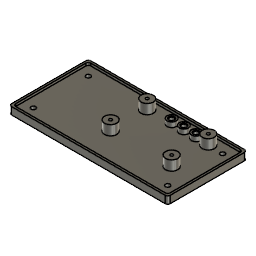
Enclosure Lid (Autodesk Fusion 360 design; units mm, degrees)
Autodesk Fusion 360 part; units mm, degrees
note: some values were not read from the file. Set by a fixed rule: the direction of a hole.
sketch "Sketch1" plane through (0, 0, 0) normal (0, 0, 1) x (1, 0, 0)
  line L0 (0, 0) -> (130, 0)
  line L1 (130, 0) -> (130, 65)
  line L2 (130, 65) -> (0, 65)
  line L3 (0, 65) -> (0, 0)
  line L4 (1.75, 1.75) -> (128.25, 1.75)
  line L5 (128.25, 1.75) -> (128.25, 63.25)
  line L6 (128.25, 63.25) -> (1.75, 63.25)
  line L7 (1.75, 63.25) -> (1.75, 1.75)
  line L8 (4, 4) -> (126, 4)
  line L9 (126, 4) -> (126, 61)
  line L10 (126, 61) -> (4, 61)
  line L11 (4, 61) -> (4, 4)
  line L12 (4, 61) -> (16, 61)
  line L13 (16, 61) -> (16, 49)
  line L14 (16, 49) -> (4, 49)
  line L15 (4, 49) -> (4, 61)
  line L16 (4, 4) -> (16, 4)
  line L17 (16, 4) -> (16, 16)
  line L18 (16, 16) -> (4, 16)
  line L19 (4, 16) -> (4, 4)
  line L20 (126, 61) -> (114, 61)
  line L21 (114, 61) -> (114, 49)
  line L22 (114, 49) -> (126, 49)
  line L23 (126, 49) -> (126, 61)
  line L24 (126, 4) -> (114, 4)
  line L25 (114, 4) -> (114, 16)
  line L26 (114, 16) -> (126, 16)
  line L27 (126, 16) -> (126, 4)
  circle A0 centre (10, 55) radius 1.75
  circle A1 centre (10, 10) radius 1.75
  circle A2 centre (120, 55) radius 1.75
  circle A3 centre (120, 10) radius 1.75
  dimension "d1" = 130
  dimension "d2" = 65
  dimension "d3" = 126.5
  dimension "d15" = 12
  dimension "d17" = 12
  dimension "d19" = 12
  dimension "d20" = 12
  dimension "d21" = 12
  dimension "d22" = 12
  dimension "d23" = 3.5
  dimension "d24" = 3.5
  dimension "d25" = 3.5
  dimension "d26" = 3.5
  dimension "d55" = 12
  dimension "d56" = 12
  dimension "d57" = 6
  dimension "d58" = 6
  dimension "d59" = 6
  dimension "d60" = 6
  dimension "d61" = 6
  dimension "d62" = 6
  dimension "d63" = 6
  dimension "d64" = 6
  dimension "d65" = 57
  dimension "d66" = 61.5
  dimension "d67" = 1.75
  dimension "d68" = 1.75
  dimension "d202" = 2.25
  dimension "d203" = 2.25
  constraint horizontal L0
  constraint vertical L1
  constraint horizontal L2
  constraint vertical L3
  constraint coincident L0.start L3.end
  constraint horizontal L4
  constraint vertical L5
  constraint horizontal L6
  constraint vertical L7
  constraint horizontal L8
  constraint vertical L9
  constraint horizontal L10
  constraint vertical L11
  constraint horizontal L12
  constraint vertical L13
  constraint horizontal L14
  constraint vertical L15
  constraint horizontal L16
  constraint vertical L17
  constraint horizontal L18
  constraint vertical L19
  constraint horizontal L20
  constraint vertical L21
  constraint horizontal L22
  constraint vertical L23
  constraint horizontal L24
  constraint vertical L25
  constraint horizontal L26
  constraint vertical L27
  measures "d1" distance of L0.start L0.end
  measures "d2" distance of L0.start L2.end
  measures "d3" distance of L4.start L4.end
  measures "d15" distance of L10.end L12.end
  measures "d17" distance of L8.start L16.end
  measures "d19" distance of L9.end L20.end
  measures "d20" distance of L9.end L22.end
  measures "d21" distance of L8.end L24.end
  measures "d22" distance of L8.end L26.end
  measures "d23" diameter of A0
  measures "d24" diameter of A1
  measures "d25" diameter of A2
  measures "d26" diameter of A3
  measures "d55" distance of L10 L14
  measures "d56" distance of L8 L18
  measures "d57" distance of L13 A0.centre
  measures "d58" distance of L10 A0.centre
  measures "d59" distance of L22 A2.centre
  measures "d60" distance of L21 A2.centre
  measures "d61" distance of L26 A3.centre
  measures "d62" distance of L25 A3.centre
  measures "d63" distance of L17 A1.centre
  measures "d64" distance of L18 A1.centre
  measures "d65" distance of L10 L16
  measures "d66" distance of L4 L6
  measures "d67" distance of L2 L6
  measures "d68" distance of L1 L5
  measures "d202" distance of L7 L11
  measures "d203" distance of L5 L23
extrude "Extrude1" add sketch "Sketch1" along normal blind 4 contours L4 L5 L6 L7 | L8 L11 L16 L17 L18 L19 | L8 L9 L10 L11 L13 L14 L17 L18 L21 L22 L25 L26 | L8 L9 L24 L25 L26 L27 | L10 L11 L12 L13 L14 L15 | L9 L10 L20 L21 L22 L23 | A0 | A1 | A2 | A3
extrude "Extrude2" add sketch "Sketch1" along normal blind 6 contours L0 L1 L2 L3
hole "Hole1" at (10, 10, 0) direction (0, 0, 1) diameter 3.75 depth 4 tip angle 118 countersink diameter 6.5 countersink angle 90
hole "Hole2" at (10, 55, 0) direction (0, 0, 1) diameter 3.75 depth 4 tip angle 118 countersink diameter 6.5 countersink angle 90
hole "Hole3" at (120, 55, 0) direction (0, 0, 1) diameter 3.75 depth 4 tip angle 118 countersink diameter 6.5 countersink angle 90
hole "Hole4" at (120, 10, 0) direction (0, 0, 1) diameter 3.75 depth 4 tip angle 118 countersink diameter 6.5 countersink angle 90
fillet "Fillet1" radius 2 1 edges at (130, 0, 3)
fillet "Fillet2" radius 2 1 edges at (1.75, 63.25, 5)
fillet "Fillet3" radius 2 1 edges at (0, 65, 3)
fillet "Fillet4" radius 2 1 edges at (128.25, 1.75, 5)
fillet "Fillet5" radius 2 1 edges at (0, 0, 3)
fillet "Fillet6" radius 2 1 edges at (128.25, 63.25, 5)
fillet "Fillet7" radius 2 1 edges at (130, 65, 3)
fillet "Fillet8" radius 2 1 edges at (1.75, 1.75, 5)
sketch "Sketch2" plane through (0, 0, 4) normal (0, 0, 1) x (-1, 0, 0)
  circle A0 centre (-120, -10) radius 1.875
  circle A1 centre (-120, -55) radius 1.875
  circle A2 centre (-10, -55) radius 1.875
  circle A3 centre (-10, -10) radius 1.875
  arc A4 (-1.75, -3.75) -> (-3.75, -1.75) centre (-3.75, -3.75) ccw
  line L0 (-3.75, -1.75) -> (-126.25, -1.75)
  arc A5 (-126.25, -1.75) -> (-128.25, -3.75) centre (-126.25, -3.75) ccw
  line L1 (-128.25, -3.75) -> (-128.25, -61.25)
  arc A6 (-128.25, -61.25) -> (-126.25, -63.25) centre (-126.25, -61.25) ccw
  line L2 (-126.25, -63.25) -> (-3.75, -63.25)
  arc A7 (-3.75, -63.25) -> (-1.75, -61.25) centre (-3.75, -61.25) ccw
  line L3 (-1.75, -61.25) -> (-1.75, -3.75)
  line L4 (-53, -60.25) -> (-113, -60.25)
  line L5 (-113, -60.25) -> (-113, -20.25)
  line L6 (-113, -20.25) -> (-53, -20.25)
  line L7 (-53, -20.25) -> (-53, -60.25)
  line L8 (-53, -50.25) -> (-53, -60.25)
  line L9 (-113, -60.25) -> (-103, -60.25)
  line L10 (-113, -50.25) -> (-113, -60.25)
  circle A8 centre (-58, -55.25) radius 1.22
  circle A9 centre (-108, -55.25) radius 1.22
  circle A10 centre (-58, -25.25) radius 1.22
  circle A11 centre (-108, -25.25) radius 1.22
  circle A12 centre (-78, -55.25) radius 1.75
  circle A13 centre (-88, -55.25) radius 1.75
  circle A14 centre (-98, -55.25) radius 1.75
  circle A15 centre (-78, -55.25) radius 3.75
  circle A16 centre (-88, -55.25) radius 3.75
  circle A17 centre (-98, -55.25) radius 3.75
  circle A18 centre (-108, -25.25) radius 5
  circle A19 centre (-58, -25.25) radius 5
  circle A20 centre (-58, -55.25) radius 5
  circle A21 centre (-108, -55.25) radius 5
  point P0 (-120, -55)
  dimension "d86" = 40
  dimension "d87" = 3
  dimension "d94" = 10
  dimension "d97" = 2.44
  dimension "d98" = 2.44
  dimension "d99" = 2.44
  dimension "d100" = 2.44
  dimension "d109" = 3.5
  dimension "d110" = 3.5
  dimension "d111" = 3.5
  dimension "d113" = 5
  dimension "d114" = 5
  dimension "d115" = 5
  dimension "d116" = 10
  dimension "d117" = 10
  dimension "d171" = 7.5
  dimension "d172" = 7.5
  dimension "d173" = 7.5
  dimension "d239" = 10
  dimension "d240" = 10
  dimension "d241" = 5
  dimension "d242" = 5
  dimension "d243" = 5
  dimension "d244" = 5
  dimension "d245" = 10
  dimension "d246" = 10
  dimension "d249" = 60
  dimension "d250" = 25
  dimension "d251" = 7
  dimension "d260" = 5
  dimension "d261" = 5
  dimension "d262" = 5
  dimension "d263" = 5
  constraint horizontal L4
  constraint vertical L5
  constraint horizontal L6
  constraint vertical L7
  constraint concentric A12 A15
  constraint concentric A13 A16
  constraint concentric A14 A17
  constraint concentric A11 A18
  constraint concentric A10 A19
  constraint concentric A8 A20
  constraint concentric A9 A21
  measures "d86" distance of L4.start L6.end
  measures "d87" distance of L2 L4
  measures "d94" distance of L4.end L10.start
  measures "d97" diameter of A8
  measures "d98" diameter of A9
  measures "d99" diameter of A10
  measures "d100" diameter of A11
  measures "d109" diameter of A12
  measures "d110" diameter of A13
  measures "d111" diameter of A14
  measures "d113" distance of L4 A12.centre
  measures "d114" distance of L4 A13.centre
  measures "d115" distance of L4 A14.centre
  measures "d116" distance of A12.centre A13.centre
  measures "d117" distance of A13.centre A14.centre
  measures "d171" diameter of A15
  measures "d172" diameter of A16
  measures "d173" diameter of A17
  measures "d239" diameter of A18
  measures "d240" diameter of A19
  measures "d241" distance of L6 A11.centre
  measures "d242" distance of L5 A11.centre
  measures "d243" distance of L7 A10.centre
  measures "d244" distance of L6 A10.centre
  measures "d245" diameter of A20
  measures "d246" diameter of A21
  measures "d249" distance of L5 L7
  measures "d250" distance of L7 A12.centre
  measures "d251" distance of P0 L5
  measures "d260" distance of L10 A9.centre
  measures "d261" distance of L4 A9.centre
  measures "d262" distance of L8 A8.centre
  measures "d263" distance of L4 A8.centre
extrude "Extrude3" add sketch "Sketch2" along normal blind 8 contours L4 L7 L8 A20 | L4 L5 L6 L7 L8 L9 L10 A18 A19 A20 A21 | A20 | L4 L5 L9 L10 A21 | A21 | L6 L7 A19 | A19 | L5 L6 A18 | A18 | A8 | A9 | A10 | A11 | A12 | A13 | A14 | A15 | A16 | A17
hole "Hole6" at (98, 55.25, 4) direction (0, 0, -1) diameter 3.1 depth 4 tip angle 118
hole "Hole7" at (88, 55.25, 4) direction (0, 0, -1) diameter 3.1 depth 4 tip angle 118
hole "Hole8" at (78, 55.25, 4) direction (0, 0, -1) diameter 3.1 depth 4 tip angle 118
sketch "Sketch3" plane through (0, 0, 0) normal (0, 0, -1) x (1, 0, 0)
  circle A0 centre (78, -55.25) radius 1.55
  circle A1 centre (88, -55.25) radius 1.55
  circle A2 centre (98, -55.25) radius 1.55
  circle A3 centre (120, -10) radius 3.25
  circle A4 centre (120, -55) radius 3.25
  circle A5 centre (10, -55) radius 3.25
  circle A6 centre (10, -10) radius 3.25
  arc A7 (128, -65) -> (130, -63) centre (128, -63) ccw
  line L0 (130, -63) -> (130, -2)
  arc A8 (130, -2) -> (128, 0) centre (128, -2) ccw
  line L1 (128, 0) -> (2, 0)
  arc A9 (2, 0) -> (0, -2) centre (2, -2) ccw
  line L2 (0, -2) -> (0, -63)
  arc A10 (0, -63) -> (2, -65) centre (2, -63) ccw
  line L3 (2, -65) -> (128, -65)
  circle A11 centre (98, -55.25) radius 1.55
  circle A12 centre (88, -55.25) radius 1.55
  circle A13 centre (88, -55.25) radius 1.55
  circle A14 centre (78, -55.25) radius 1.55
  line L4 (86.5, -39.5293) -> (86.5, -50.25) construction
  line L5 (86.5, -50.25) -> (89.5, -50.25) construction
  line L6 (89.5, -50.25) -> (89.5, -39.5293) construction
  line L7 (89.5, -39.5293) -> (86.5, -39.5293) construction
  line L8 (96, -35.4684) -> (96, -50.25) construction
  line L9 (96, -50.25) -> (100, -50.25) construction
  line L10 (100, -50.25) -> (100, -35.4684) construction
  line L11 (100, -35.4684) -> (96, -35.4684) construction
  line L12 (76.5, -40.1241) -> (76.5, -50.25) construction
  line L13 (76.5, -50.25) -> (79.5, -50.25) construction
  line L14 (79.5, -50.25) -> (79.5, -40.1241) construction
  line L15 (79.5, -40.1241) -> (76.5, -40.1241) construction
  line L16 (29.4817, -12.6071) -> (114.991, -12.7409) construction
  line L17 (114.991, -12.7409) -> (115.009, -1.2591) construction
  line L18 (115.009, -1.2591) -> (29.4997, -1.1254) construction
  line L19 (29.4997, -1.1254) -> (29.4817, -12.6071) construction
  line L20 (36.9967, -17.8385) -> (115.0014, -17.7991) construction
  line L21 (115.0014, -17.7991) -> (114.9986, -12.2009) construction
  line L22 (114.9986, -12.2009) -> (36.9939, -12.2403) construction
  line L23 (36.9939, -12.2403) -> (36.9967, -17.8385) construction
  dimension "d134" = 3.1
  dimension "d135" = 3.1
  dimension "d136" = 3.1
  dimension "d177" = 4
  dimension "d178" = 4
  dimension "d179" = 4
  dimension "d180" = 5
  dimension "d181" = 5
  dimension "d182" = 5
  dimension "d183" = 32
  dimension "d184" = 10
  dimension "d185" = 10
  dimension "d204" = 7
  dimension "d205" = 3
  dimension "d235" = 15
  dimension "d236" = 15
  dimension "d237" = 7
  dimension "d238" = 15
  constraint concentric A2 A11
  constraint concentric A1 A12
  constraint concentric A12 A13
  constraint concentric A0 A14
  measures "d134" diameter of A11
  measures "d135" diameter of A13
  measures "d136" diameter of A14
  measures "d180" distance of A2.centre
  measures "d181" distance of A1.centre
  measures "d182" distance of A0.centre
emboss "Emboss5" [suppressed]
extrude "Extrude5" add sketch "Sketch2" along normal blind 5.2 contours A15 | A16 | A17
hole "Hole12" at (78, 55.25, 0) direction (0, 0, 1) diameter 3.5 depth 11 tip angle 118 countersink diameter 6 countersink angle 90
hole "Hole13" at (88, 55.25, 0) direction (0, 0, 1) diameter 3.5 depth 11 tip angle 118 countersink diameter 6 countersink angle 90
hole "Hole14" at (98, 55.25, 0) direction (0, 0, 1) diameter 3.5 depth 11 tip angle 118 countersink diameter 6 countersink angle 90
extrude "Extrude6" add sketch "Sketch2" along normal blind 8 contours A20 | A21 | A19 | A18
extrude "Extrude7" cut 1 faces at (84.6667, 31.8881, 12) along direction (0, 0, -1) blind 8
extrude "Extrude8" add sketch "Sketch2" along normal blind 8 contours A20 | A21 | A19 | A18
extrude "Extrude9" add sketch "Sketch2" along normal blind 5 contours A15 | A16 | A17
sketch "Sketch4" plane through (130, 0, 0) normal (1, 0, 0) x (0, 1, 0)
  line L0 (63, 0) -> (63, 6)
  line L1 (63, 6) -> (2, 6)
  line L2 (2, 6) -> (2, 0)
  line L3 (2, 0) -> (63, 0)
extrude "Extrude10" cut 1 faces at (107.0908, 55.1894, 4) along direction (0, 0, -1) blind 1
extrude "Extrude11" cut 1 faces at (57.2071, 55.5133, 4) along direction (0, 0, -1) blind 1
extrude "Extrude12" cut 1 faces at (58.336, 25.4791, 4) along direction (0, 0, -1) blind 1
extrude "Extrude13" cut 1 faces at (108.1486, 25.7498, 4) along direction (0, 0, -1) blind 1
extrude "Extrude14" cut 3 faces at (94.9306, 55.4363, 9) (84.9306, 55.4363, 9) (74.9306, 55.4363, 9) along direction (0, 0, -1) blind 1
move_face "OffsetFaces1" offset -0.125 2 faces at (98, 57, 6.6667) (96.25, 55.25, 2.1667)
move_face "OffsetFaces2" offset -0.125 2 faces at (88, 57, 6.6667) (86.25, 55.25, 2.1667)
move_face "OffsetFaces3" offset -0.125 2 faces at (78, 57, 6.6667) (76.25, 55.25, 2.1667)
chamfer "Chamfer1" distance 0.5 angle 45 1 edges at (99.7481, 55.928, 8)
chamfer "Chamfer2" distance 0.5 angle 45 1 edges at (89.7481, 55.928, 8)
chamfer "Chamfer3" distance 0.5 angle 45 1 edges at (79.7481, 55.928, 8)
hole "Hole9" [suppressed]
hole "Hole10" [suppressed]
hole "Hole11" [suppressed]
fillet "Fillet9" [suppressed]
fillet "Fillet10" [suppressed]
fillet "Fillet11" [suppressed]
fillet "Fillet12" [suppressed]
fillet "Fillet13" [suppressed]
fillet "Fillet14" [suppressed]
fillet "Fillet15" [suppressed]
fillet "Fillet16" [suppressed]
fillet "Fillet17" [suppressed]
extrude "Extrude4" [suppressed]
emboss "Emboss4" [suppressed]
